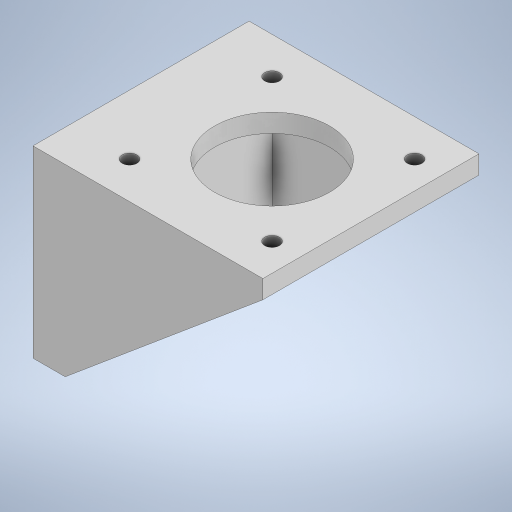
# Autodesk Inventor part: Extruder Mount
Saved by Autodesk Inventor 2023.1 (Build 271208000, 208)
## iProperties
Created: 2022-11-07
Part Number: Extruder Mount
Material: Generic
Document SubType Name: Modeling
Designer: nicol
Density: 1 g/cm^3
Appearance: Default
Author: nicol
Autodesk Inventor part; units mm, degrees
ref_plane "YZ Plane" through (0, 0, 0) normal (1, 0, 0) x (0, 1, 0)
ref_plane "XZ Plane" through (0, 0, 0) normal (0, 1, 0) x (-1, 0, 0)
ref_plane "XY Plane" through (0, 0, 0) normal (0, 0, 1) x (1, 0, 0)
sketch "Sketch1" plane through (0, 0, 0) normal (0, 0, 1) x (1, 0, 0)
  line L0 (0, 0) -> (0, 40)
  line L1 (0, 40) -> (50, 40)
  line L2 (50, 40) -> (50, 36)
  line L3 (50, 36) -> (7, 36)
  line L4 (7, 36) -> (7, 0)
  line L5 (7, 0) -> (0, 0)
  dimension "d0" = 40
  dimension "d1" = 43
  dimension "d2" = 4
  dimension "d3" = 7
  constraints: 12 end point, 4 perpendicular, 1 horizontal, 1 vertical
  measures "d0" distance of L0.start L0.end
  measures "d1" distance of L2.end L3.end
  measures "d2" distance of L1.end L2.end
  measures "d3" distance of L4.end L0.start
extrude "Extrusion1" add sketch "Sketch1" along normal blind 43
sketch "Sketch2" plane through (0, 0, 43) normal (0, 0, 1) x (1, 0, 0)
  line L0 (7, 0) -> (7, 36) projected
  line L1 (7, 36) -> (50, 36) projected
  line L2 (50, 36) -> (50, 40) projected
  line L3 (50, 40) -> (0, 40) projected
  line L4 (0, 40) -> (0, 0) projected
  line L5 (0, 0) -> (7, 0) projected
  line L6 (7, 0) -> (7, 36) projected
  line L7 (7, 36) -> (50, 36) projected
  line L8 (7, 0) -> (50, 36)
  constraints: 2 end point
extrude "Extrusion2" add sketch "Sketch2" along normal blind 2
sketch "Sketch3" plane through (0, 0, 0) normal (0, 0, -1) x (-1, 0, 0)
  line L0 (-7, 0) -> (-7, 36) projected
  line L1 (0, 0) -> (-7, 0) projected
  line L2 (0, 40) -> (0, 0) projected
  line L3 (-50, 40) -> (0, 40) projected
  line L4 (-50, 36) -> (-50, 40) projected
  line L5 (-7, 36) -> (-50, 36) projected
  line L6 (0, 0) -> (-7, 0) projected
  line L7 (-7, 0) -> (-50, 36) projected
  line L8 (-7, 0) -> (-50, 36)
  constraints: 2 end point, 1 collinear
extrude "Extrusion3" add sketch "Sketch3" along normal blind 2
sketch "Sketch4" plane through (7, 36, 43) normal (0, -1, 0) x (1, 0, 0)
  line L0 (0, -43) -> (43, -43) projected
  line L1 (43, -43) -> (43, 0) projected
  line L2 (0, 0) -> (43, 0) projected
  line L3 (0, -43) -> (0, 0) projected
  line L4 (37, -6) -> (6, -6) construction
  line L5 (6, -6) -> (6, -37) construction
  line L6 (6, -37) -> (37, -37) construction
  line L7 (37, -37) -> (37, -6) construction
  line L8 (0, 0) -> (43, 0) construction
  point P0 (-7, -43)
  point P1 (21.5, -21.5)
  point P2 (37, -21.5)
  point P3 (43, -21.5)
  point P4 (21.5, 0)
  point P5 (21.5, -6)
  dimension "d10" = 31
  dimension "d11" = 31
  constraints: 8 end point, 4 coincident, 4 midpoint, 2 horizontal alignment, 2 parallel, 2 vertical alignment, 1 horizontal, 1 perpendicular
  measures "d10" distance of L4.start L4.end
  measures "d11" distance of L6.end L4.start
hole "Hole1" at (44, 36, 37) at (44, 36, 6) at (13, 36, 6) at (13, 36, 37) direction (0, 1, 0) diameter 3.2 end through all
hole "Hole2" at (28.5, 36, 21.5) direction (0, 1, 0) diameter 25 end through all
sketch "Sketch5" plane through (0, 0, 45) normal (-1, 0, 0) x (0, 0, 1)
  line L0 (-47, 40) -> (0, 40) projected
  line L1 (-47, 0) -> (0, 0) projected
  point P0 (-45, 0)
  point P1 (-23.5, 30)
  point P2 (-23.5, 10)
  point P3 (-23.5, 40)
  dimension "d26" = 10
  dimension "d27" = 10
  constraints: 2 vertical alignment, 1 midpoint
  measures "d26" distance from line of point (-23.5, 30) L0
  measures "d27" distance from line of L1 point (-23.5, 10)
hole "Hole3" at (0, 30, 21.5) at (0, 10, 21.5) direction (1, 0, 0) diameter 5.2 end through all
sketch "Sketch6" plane through (7, 0, 43) normal (1, 0, 0) x (0, 0, -1)
  circle A0 centre (21.5, 30) radius 2.6 projected
  circle A1 centre (21.5, 10) radius 2.6 projected
  line L0 (43, 0) -> (43, 36) projected
  line L1 (43, 36) -> (0, 36) projected
  line L2 (0, 0) -> (0, 36) projected
  line L3 (43, 0) -> (0, 0) projected
  circle A2 centre (21.5, 30) radius 5
  circle A3 centre (21.5, 10) radius 5
  point P0 (43, 0)
  dimension "d35" = 10
  dimension "d36" = 10
  constraints: 2 centre point, 2 coincident
  measures "d35" diameter of A2
  measures "d36" diameter of A3
extrude "Extrusion4" cut sketch "Sketch6" against normal blind 3 contours A2 | A3
body "Solid1"
